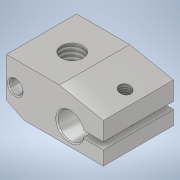
# Autodesk Inventor part: MINI-heaterblock
Saved by Autodesk Inventor 2021 (Build 250183000, 183)
## iProperties
Company: Prusa Development a.s.
Created: 2019-02-15
Material: Všeobecné
Document SubType Name: Modeling
Density: 1 g/cm^3
Appearance: Hliník – tmavý
Project: ORIGINAL PRUSA MINI
Authority: Ing. Robert Turinský
Author: Ing. Robert Turinský
Title: MINI-heaterblock
Revision Number: R4
Autodesk Inventor part; units mm, degrees
ref_plane "YZ Plane" through (0, 0, 0) normal (1, 0, 0) x (0, 1, 0)
ref_plane "XZ Plane" through (0, 0, 0) normal (0, 1, 0) x (-1, 0, 0)
ref_plane "XY Plane" through (0, 0, 0) normal (0, 0, 1) x (1, 0, 0)
sketch "Náčrt1" plane through (0, 0, 0) normal (0, 0, 1) x (1, 0, 0)
  line L0 (3.85, 5.5) -> (-3, 5.5)
  line L1 (-7, 1.5) -> (-7, -1.5)
  line L2 (-3, -5.5) -> (8.1, -5.5)
  line L3 (0, -7.9925) -> (0, 9.4552) projected
  line L4 (-11.42, 0) -> (19.52, 0) projected
  arc A0 (10.3914, -0.7) -> (10.3914, -2.3) centre (7.5, -1.5) ccw
  line L5 (15.1, -0.7) -> (10.3914, -0.7)
  line L6 (10.3914, -2.3) -> (15.1, -2.3)
  line L7 (15.1, -3.3) -> (15.1, -2.3)
  line L8 (15.1, -0.7) -> (15.1, 1.3)
  circle A1 centre (-5, 0) radius 1.55
  line L9 (15.1, 1.3) -> (9.8482, 1.3)
  line L10 (9.8482, 1.3) -> (3.85, 5.5)
  line L11 (15.1, -3.3) -> (8.1, -5.5)
  line L12 (0, 5.5) -> (0, 6.9627)
  line L13 (10.3914, -2.3) -> (15.1, -2.3)
  line L14 (15.1, -2.3) -> (15.1, -3.3)
  line L15 (8.1, -5.5) -> (15.1, -3.3)
  line L16 (8.1, -5.5) -> (-3, -5.5)
  line L17 (-7, -1.5) -> (-7, 1.5)
  line L18 (-3, 5.5) -> (3.85, 5.5)
  line L19 (3.85, 5.5) -> (9.8482, 1.3)
  line L20 (9.8482, 1.3) -> (15.1, 1.3)
  line L21 (15.1, 1.3) -> (15.1, -0.7)
  line L22 (15.1, -0.7) -> (10.3914, -0.7)
  line L23 (0, 5.5) -> (-2.5, 5.5)
  line L24 (-2.5, 5.5) -> (-2.5, -5.5)
  line L25 (-2.5, -5.5) -> (0, -5.5)
  line L26 (0, -5.5) -> (0, 5.5)
  line L27 (0, 5.5) -> (-2.5, 5.5)
  line L28 (-2.5, 5.5) -> (-2.5, -5.5)
  line L29 (-2.5, -5.5) -> (0, -5.5)
  line L30 (0, -5.5) -> (0, 5.5)
  line L31 (13.35, 1.3) -> (12.05, 1.3)
  line L32 (12.05, 1.3) -> (12.05, -1.5)
  line L33 (12.05, -1.5) -> (13.35, -1.5)
  line L34 (13.35, -1.5) -> (13.35, 1.3)
  line L35 (12.05, -1.5) -> (13.6, -1.5)
  line L36 (13.6, -1.5) -> (13.6, -5.5)
  line L37 (13.6, -5.5) -> (12.05, -5.5)
  line L38 (12.05, -5.5) -> (12.05, -1.5)
  line L39 (-5, 0) -> (-6.25, 0)
  line L40 (-6.25, 0) -> (-6.25, -5.5)
  line L41 (-6.25, -5.5) -> (-5, -5.5)
  line L42 (-5, -5.5) -> (-5, 0)
  line L43 (15.1, -3.3) -> (13.6, -3.3)
  line L44 (13.6, -3.3) -> (13.6, -5.5)
  line L45 (13.6, -5.5) -> (15.1, -5.5)
  line L46 (15.1, -5.5) -> (15.1, -3.3)
  line L47 (-6.25, -5.5) -> (-7, -5.5)
  line L48 (-7, -5.5) -> (-7, -1.5)
  line L49 (-7, -1.5) -> (-6.25, -1.5)
  line L50 (-6.25, -1.5) -> (-6.25, -5.5)
  line L51 (-6.25, 0) -> (-5, 0)
  line L52 (-5, 0) -> (-5, -5.5)
  line L53 (-5, -5.5) -> (-6.25, -5.5)
  line L54 (-6.25, -5.5) -> (-6.25, 0)
  line L55 (15.1, 1.3) -> (15.1, 5.5)
  line L56 (15.1, 5.5) -> (3.85, 5.5)
  line L57 (-3, 5.5) -> (-7, 5.5)
  line L58 (-7, 5.5) -> (-7, 1.5)
  line L59 (13.35, -1.5) -> (12.05, -1.5)
  line L60 (12.05, -1.5) -> (12.05, 5.5)
  line L61 (12.05, 5.5) -> (13.35, 5.5)
  line L62 (13.35, 5.5) -> (13.35, -1.5)
  line L63 (-7, -1.5) -> (-7, -3.5)
  line L64 (-3, -5.5) -> (-7, -3.5)
  line L65 (15.1, -3.3) -> (15.1, -5.5)
  line L66 (15.1, -5.5) -> (8.1, -5.5)
  point P0 (15.1, 0)
  point P1 (-7, 0)
  dimension "d2" = 6
  dimension "d3" = 1.6
  dimension "d4" = 4
  dimension "d5" = 14.5
  dimension "d6" = 3.1
  dimension "d7" = 2
  dimension "d8" = 7
  dimension "d9" = 11
  dimension "d10" = 2
  dimension "d11" = 22.1
  dimension "d15" = 1
  dimension "d18" = 5
  dimension "d20" = 3.05
  dimension "d21" = 2.6
  dimension "d22" = 3.1
  dimension "d23" = 2.5
  dimension "d59" = 7
  dimension "d67" = 4
  dimension "d68" = 35
  dimension "d79" = 3.85
  dimension "d88" = 4
  dimension "d89" = 2
  dimension "d90" = 1.5
  constraints: 130 end point, 23 parallel, 14 perpendicular, 13 horizontal, 12 collinear, 10 point on line, 3 vertical, 2 centre point, 2 midpoint, 2 point on circle, 1 other
  measures "d2" diameter of A0
  measures "d3" distance between parallel lines of L6 L5
  measures "d4" distance from line of A0.centre L2
  measures "d5" distance from line of L1 A0.centre
  measures "d6" diameter of A1
  measures "d7" distance from line of L1 L39.start
  measures "d8" distance from line of L1 L12.start
  measures "d9" distance between parallel lines of L2 L0
  measures "d10" distance between parallel lines of L9 L5
  measures "d11" distance between parallel lines of L1 L8
  measures "d15" distance from line of L6 L7.start
  measures "d18" diameter of L24 L26
  measures "d20" distance between parallel lines of L8 L32
  measures "d21" diameter of L34 L32
  measures "d22" diameter of L36 L38
  measures "d23" diameter of L40 L42
  measures "d59" horizontal distance of L2.end L7.start
  measures "d67" horizontal distance of L1.start L0.end
  measures "d68" angle of L0 L10
  measures "d79" distance from line of L3 L0.start
  measures "d88" horizontal distance of L2.start L63.end
  measures "d89" vertical distance of L2.start L63.end
  measures "d90" distance between parallel lines of L4 L49
extrude "Vysunutí1" add sketch "Náčrt1" along normal mid plane 16 contours L10 L9 L32 L4 A0 L3 L0 | L56 L60 L9 L10 | L3 L4 L24 L0 | L56 L62 L9 L60 | L24 L4 A1 L1 L58 L57 L0 | L4 A0 L6 L38 L11 L2 L3 | L3 L2 L24 L4 | L9 L34 L4 L32 | L56 L55 L9 L62 | L24 L2 L64 L42 A1 L4 | L9 L8 L4 L34 | L32 L5 A0 L4 | L4 L34 L5 L32 | L11 L38 L66 | L4 L8 L5 L34 | A1 L40 L49 L1 L4 | L42 L64 L40 A1 | L38 L6 L36 L11 | L11 L36 L37 L38 | L36 L43 L11 | L11 L46 L45 L36 | L6 L7 L43 L36 | L49 L40 L64 L48
revolve "Rotace1" cut sketch "Náčrt1" angle 360 about axis through (0, -5.5, 0) along (0, 1, 0) contours L3 L4 L24 L0 | L3 L2 L24 L4
revolve "Rotace3" cut sketch "Náčrt1" angle 360 about axis through (12.05, 1.3, 0) along (0, -1, 0) contours L56 L62 L9 L60 | L9 L34 L4 L32 | L4 L34 L5 L32 | L5 L34 L33 L32 | L38 L6 L36 L11 | L11 L36 L37 L38 | L38 L33 L35 L36 L6
revolve "Rotace5" cut sketch "Náčrt1" angle 360 about axis through (-5, 0, 0) along (0, -1, 0) contours L42 A1 L40 L4 | L42 L64 L40 A1 | L42 L41 L40 L64
thread "Závit3" size "M6x1" class "6H" standard "ANSI Metric M Profile" full length
thread "Závit5" size "M3x0.5" class "6H" standard "ANSI Metric M Profile" full length
chamfer "Zkosení1" distance 0.25 angle 45 4 edges at (4.5, -1.5, -8) (4.5, -1.5, 8) (-6.55, 0, -8) (-6.55, 0, 8)
chamfer "Zkosení2" distance 0.6 angle 45 1 edges at (2.5, -5.5, 0)
chamfer "Zkosení5" distance 2 distance2 10 1 edges at (15.1, 5.5, 0)
thread "Závit6" size "M3x0.5" class "6H" standard "ANSI Metric M Profile" full length
